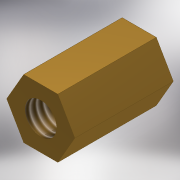
# Autodesk Inventor part: StandoffM4x10A
Saved by Autodesk Inventor 2018 (Build 220112000, 112)
## iProperties
Created: 2018-03-25
Part Number: StandoffM4x10A
Material: Brass, Soft Yellow
Document SubType Name: Modeling
Designer: mansu
Density: 8.47 g/cm^3
Appearance: Brass - Satin
Author: mansu
Autodesk Inventor part; units mm, degrees
ref_plane "YZ Plane" through (0, 0, 0) normal (1, 0, 0) x (0, 1, 0)
ref_plane "XZ Plane" through (0, 0, 0) normal (0, 1, 0) x (-1, 0, 0)
ref_plane "XY Plane" through (0, 0, 0) normal (0, 0, 1) x (1, 0, 0)
sketch "Sketch1" plane through (0, 0, 0) normal (0, 1, 0) x (-1, 0, 0)
  line L0 (-1.7321, -3) -> (-3.4641, 0)
  line L1 (-3.4641, 0) -> (-1.7321, 3)
  line L2 (-1.7321, 3) -> (1.7321, 3)
  line L3 (1.7321, 3) -> (3.4641, 0)
  line L4 (3.4641, 0) -> (1.7321, -3)
  line L5 (1.7321, -3) -> (-1.7321, -3)
  point P0 (0, 0)
  point P1 (0, 0)
  dimension "d0" = 3
  constraints: 12 end point, 1 coincident, 13 other
  measures "d0" distance from line of L5 point (0, 0)
extrude "Extrusion1" add sketch "Sketch1" along normal blind 10
sketch "Sketch2" plane through (0, 10, 0) normal (0, 1, 0) x (1, 0, 0)
  point P0 (0, 0)
hole "Hole1" at (0, 10, 0) direction (0, -1, 0) diameter 3.242 end through all thread size "M4x0.7" class "6H" standard "ISO Metric profile"
body "Solid1"
